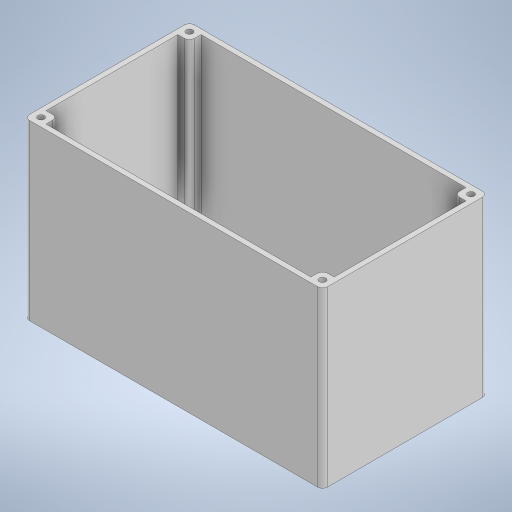
# Autodesk Inventor part: box_bottom
Saved by Autodesk Inventor 2024.2 (Build 282272000, 272)
## iProperties
Created: 2025-03-01
Part Number: box_bottom
Material: Všeobecné
Document SubType Name: Modeling
Designer: hepma_axt67em
Density: 1 g/cm^3
Appearance: Výchozí
Author: hepma_axt67em
Autodesk Inventor part; units mm, degrees
ref_plane "YZ Plane" through (0, 0, 0) normal (1, 0, 0) x (0, 1, 0)
ref_plane "XZ Plane" through (0, 0, 0) normal (0, 1, 0) x (-1, 0, 0)
ref_plane "XY Plane" through (0, 0, 0) normal (0, 0, 1) x (1, 0, 0)
sketch "Náčrt1" plane through (0, 0, 0) normal (0, 1, 0) x (-1, 0, 0)
  line L0 (0, -68.6) -> (0, 68.6) projected
  line L1 (-123.9, 0) -> (123.9, 0) projected
  line L2 (88.5, -49) -> (-88.5, -49)
  line L3 (-88.5, -49) -> (-88.5, 49)
  line L4 (-88.5, 49) -> (88.5, 49)
  line L5 (88.5, 49) -> (88.5, -49)
  point P0 (0, 0)
  dimension "d0" = 98
  dimension "d1" = 177
  constraints: 8 end point, 2 parallel, 1 horizontal, 1 perpendicular, 2 other
  measures "d0" distance of L2.end L3.end
  measures "d1" distance of L3.end L4.end
extrude "Vysunutí1" add sketch "Náčrt1" along normal blind 3
sketch "Náčrt2" plane through (0, 3, 0) normal (0, 1, 0) x (1, 0, 0)
  line L0 (88.5, 49) -> (-88.5, 49) projected
  line L1 (-88.5, 49) -> (-88.5, -49) projected
  line L2 (-88.5, -49) -> (88.5, -49) projected
  line L3 (88.5, -49) -> (88.5, 49) projected
  line L4 (88.5, 49) -> (-88.5, 49) projected
  line L5 (-88.5, 49) -> (-88.5, -49) projected
  line L6 (-88.5, 49) -> (88.5, 49)
  line L7 (88.5, 49) -> (88.5, -49)
  line L8 (88.5, -49) -> (-88.5, -49)
  line L9 (-88.5, -49) -> (-88.5, 49)
  line L10 (-85.5, -39.1) -> (-85.5, 39.1)
  line L11 (-85.5, 39.1) -> (-78.6, 39.1)
  line L12 (-78.6, 39.1) -> (-78.6, 46)
  line L13 (-78.6, 46) -> (78.6, 46)
  line L14 (78.6, 46) -> (78.6, 39.1)
  line L15 (78.6, 39.1) -> (85.5, 39.1)
  line L16 (85.5, 39.1) -> (85.5, -39.1)
  line L17 (85.5, -39.1) -> (78.6, -39.1)
  line L18 (78.6, -39.1) -> (78.6, -46)
  line L19 (78.6, -46) -> (-78.6, -46)
  line L20 (-78.6, -46) -> (-78.6, -39.1)
  line L21 (-78.6, -39.1) -> (-85.5, -39.1)
  point P0 (0, 0)
  dimension "d4" = 3
  dimension "d5" = 3
  dimension "d6" = 3
  dimension "d7" = 3
  dimension "d8" = 9.9
  dimension "d9" = 9.9
  dimension "d10" = 9.9
  dimension "d11" = 9.9
  dimension "d12" = 9.9
  dimension "d13" = 9.9
  dimension "d14" = 9.9
  dimension "d15" = 9.9
  constraints: 32 end point, 7 perpendicular, 6 parallel, 2 horizontal, 1 collinear
  measures "d4" distance between parallel lines of L1 L10
  measures "d5" distance between parallel lines of L0 L13
  measures "d6" distance between parallel lines of L7 L16
  measures "d7" distance between parallel lines of L8 L19
  measures "d8" distance between parallel lines of L1 L12
  measures "d9" distance between parallel lines of L0 L11
  measures "d10" distance between parallel lines of L8 L21
  measures "d11" distance between parallel lines of L9 L20
  measures "d12" distance between parallel lines of L7 L18
  measures "d13" distance between parallel lines of L8 L17
  measures "d14" distance between parallel lines of L0 L15
  measures "d15" distance between parallel lines of L7 L14
extrude "Vysunutí2" add sketch "Náčrt2" along normal blind 100
fillet "Zaoblení1" radius 3 8 edges at (-78.6, 53, -39.1) (78.6, 53, -39.1) (-78.6, 53, 39.1) (78.6, 53, 39.1) (88.5, 51.5, -49) (-88.5, 51.5, -49) (-88.5, 51.5, 49) (88.5, 51.5, 49)
sketch "Náčrt3" plane through (0, 103, 0) normal (0, 1, 0) x (1, 0, 0)
  line L0 (-88.5, 49) -> (-88.5, -49) projected
  line L1 (85.5, 49) -> (-85.5, 49) projected
  line L2 (-88.5, 46) -> (-88.5, -46) projected
  line L3 (-85.5, -49) -> (85.5, -49) projected
  line L4 (88.5, -46) -> (88.5, 46) projected
  arc A0 (81.6, -39.1) -> (78.6, -42.1) centre (81.6, -42.1) ccw projected
  line L5 (78.6, -42.1) -> (78.6, -46) projected
  line L6 (78.6, -46) -> (-78.6, -46) projected
  line L7 (-78.6, -46) -> (-78.6, -42.1) projected
  arc A1 (-78.6, -42.1) -> (-81.6, -39.1) centre (-81.6, -42.1) ccw projected
  line L8 (-81.6, -39.1) -> (-85.5, -39.1) projected
  line L9 (-85.5, -39.1) -> (-85.5, 39.1) projected
  line L10 (-85.5, 39.1) -> (-81.6, 39.1) projected
  arc A2 (-81.6, 39.1) -> (-78.6, 42.1) centre (-81.6, 42.1) ccw projected
  line L11 (-78.6, 42.1) -> (-78.6, 46) projected
  line L12 (-78.6, 46) -> (78.6, 46) projected
  line L13 (78.6, 46) -> (78.6, 42.1) projected
  arc A3 (78.6, 42.1) -> (81.6, 39.1) centre (81.6, 42.1) ccw projected
  line L14 (81.6, 39.1) -> (85.5, 39.1) projected
  line L15 (85.5, 39.1) -> (85.5, -39.1) projected
  line L16 (85.5, -39.1) -> (81.6, -39.1) projected
  arc A4 (85.5, -49) -> (88.5, -46) centre (85.5, -46) ccw projected
  arc A5 (88.5, 46) -> (85.5, 49) centre (85.5, 46) ccw projected
  arc A6 (-85.5, 49) -> (-88.5, 46) centre (-85.5, 46) ccw projected
  arc A7 (-88.5, -46) -> (-85.5, -49) centre (-85.5, -46) ccw projected
  point P0 (0, 0)
  point P1 (-83.55, 44.05)
  point P2 (-83.55, -44.05)
  point P3 (83.55, -44.05)
  point P4 (83.55, 44.05)
  dimension "d19" = 4.95
  dimension "d20" = 4.95
  dimension "d21" = 4.95
  dimension "d22" = 4.95
  dimension "d23" = 4.95
  dimension "d24" = 4.95
  dimension "d25" = 4.95
  dimension "d26" = 4.95
  measures "d19" distance from line of L1 point (-83.55, 44.05)
  measures "d20" distance from line of L0 point (-83.55, 44.05)
  measures "d21" distance from line of L3 point (-83.55, -44.05)
  measures "d22" distance from line of L0 point (-83.55, -44.05)
  measures "d23" distance from line of L4 point (83.55, -44.05)
  measures "d24" distance from line of L3 point (83.55, -44.05)
  measures "d25" distance from line of L4 point (83.55, 44.05)
  measures "d26" distance from line of L1 point (83.55, 44.05)
hole "Díra1" at (-83.55, 103, -44.05) at (-83.55, 103, 44.05) at (83.55, 103, 44.05) at (83.55, 103, -44.05) direction (0, -1, 0) diameter 3.9 depth 60
sketch "Náčrt4" plane through (0, 3, 0) normal (0, 1, 0) x (1, 0, 0)
  line L0 (0, 68.6) -> (0, -68.6) projected
  line L1 (123.9, 0) -> (-123.9, 0) projected
  line L2 (85.5, 39.1) -> (85.5, -39.1) projected
  point P0 (0, 0)
  point P1 (-18.5, 25.5)
  point P2 (77.5, 25.5)
  point P3 (-18.5, -25.5)
  point P4 (77.5, -25.5)
  dimension "d34" = 51
  dimension "d35" = 96
  dimension "d36" = 96
  dimension "d37" = 51
  dimension "d38" = 8
  dimension "d39" = 25.5
  constraints: 1 symmetric about line
  measures "d34" distance of point (-18.5, -25.5) point (-18.5, 25.5)
  measures "d35" distance of point (77.5, 25.5) point (-18.5, 25.5)
  measures "d36" distance of point (77.5, -25.5) point (-18.5, -25.5)
  measures "d37" distance of point (77.5, 25.5) point (77.5, -25.5)
  measures "d38" distance from line of L2 point (77.5, -25.5)
  measures "d39" distance from line of L1 point (77.5, -25.5)
hole "Díra2" at (-18.5, 3, -25.5) at (77.5, 3, -25.5) at (-18.5, 3, 25.5) at (77.5, 3, 25.5) direction (0, -1, 0) diameter 3.4 end through all clearance for "Šroub se zápustnou hlavou ISO 2009/7046" size "M3" standard "ISO"
sketch "Náčrt5" plane through (0, 3, 0) normal (0, 1, 0) x (1, 0, 0)
  line L0 (-85.5, -39.1) -> (-85.5, 39.1) projected
  line L1 (123.9, 0) -> (-123.9, 0) projected
  line L2 (-74, -38) -> (-33, -38)
  line L3 (-33, -38) -> (-33, 38)
  line L4 (-33, 38) -> (-74, 38)
  line L5 (-74, 38) -> (-74, -38)
  circle A0 centre (-18.5, 25.5) radius 1.7 projected
  point P0 (0, 0)
  dimension "d47" = 41
  dimension "d48" = 76
  dimension "d49" = 14.5
  constraints: 8 end point, 2 parallel, 1 horizontal, 1 perpendicular, 1 other
  measures "d47" distance of L3.end L4.end
  measures "d48" distance of L2.end L3.end
  measures "d49" distance from line of L3 A0.centre
extrude "Vysunutí3" cut sketch "Náčrt5" against normal blind 1 contours L3 L2 L5 L1 | L1 L5 L4 L3
chamfer "Zkosení1" distance 1.5 angle 45 4 edges at (77.5, 0, -27.2) (77.5, 0, 23.8) (-18.5, 0, -27.2) (-18.5, 0, 23.8)
sketch "Náčrt6" plane through (-88.5, 0, -46) normal (-1, 0, 0) x (0, 0, 1)
  line L0 (-22.6, 0) -> (114.6, 0) projected
  line L1 (46, 123.6) -> (46, -20.6) projected
  point P0 (46, 0)
  point P1 (46, 35)
  dimension "d55" = 35
  constraints: 1 point on line
  measures "d55" distance from line of L0 point (46, 35)
hole "Díra3" at (-88.5, 35, 0) direction (1, 0, 0) diameter 15.2 depth 3 tip angle 118
equation "\"d9\" = d8"
equation "\"d10\" = d8"
equation "\"d11\" = d8"
equation "\"d12\" = d8"
equation "\"d13\" = d8"
equation "\"d14\" = d8"
equation "\"d15\" = d8"
equation "\"d19\" = 0.5 * d8"
equation "\"d20\" = d19"
equation "\"d21\" = d20"
equation "\"d22\" = d19"
equation "\"d23\" = d22"
equation "\"d24\" = d21"
equation "\"d25\" = d19"
equation "\"d26\" = d19"
